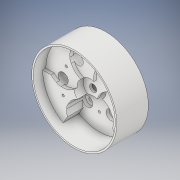
# Autodesk Inventor part: Base
Saved by Autodesk Inventor 2017 SP1 (Build 210196100, 196)
## iProperties
Created: 2017-09-22
Part Number: Base
Material: ABS Plastic
Document SubType Name: Modeling
Designer: Zach
Density: 1.06 g/cm^3
Appearance: CR White
Author: Zach
Autodesk Inventor part; units mm, degrees
ref_plane "YZ Plane" through (0, 0, 0) normal (1, 0, 0) x (0, 1, 0)
ref_plane "XZ Plane" through (0, 0, 0) normal (0, 1, 0) x (-1, 0, 0)
ref_plane "XY Plane" through (0, 0, 0) normal (0, 0, 1) x (1, 0, 0)
sketch "Sketch1" plane through (0, 0, 0) normal (0, 0, 1) x (1, 0, 0)
  circle A0 centre (0, 0) radius 54
  dimension "d0" = 108
  constraints: 1 centre point, 1 coincident
  measures "d0" diameter of A0
extrude "Extrusion1" add sketch "Sketch1" along normal blind 37
sketch "Sketch2" plane through (0, 0, 37) normal (0, 0, 1) x (1, 0, 0)
  circle A0 centre (0, 0) radius 54 projected
  circle A1 centre (0, 0) radius 52
  dimension "d3" = 2
  constraints: 1 centre point
  measures "d3" radial gap between concentric circles of A0 A1
extrude "Extrusion2" cut sketch "Sketch2" against normal blind 29 contours A1
sketch "Sketch3" plane through (0, 0, 8) normal (0, 0, 1) x (1, 0, 0)
  circle A0 centre (0, 0) radius 11
  dimension "d6" = 22
  constraints: 1 centre point, 1 coincident
  measures "d6" diameter of A0
extrude "Extrusion3" cut sketch "Sketch3" against normal through all
sketch "Sketch4" plane through (0, 0, 8) normal (0, 0, 1) x (1, 0, 0)
  circle A0 centre (30, 0) radius 6.5
  circle A1 centre (15, 25.9808) radius 6.5
  circle A2 centre (-15, 25.9808) radius 6.5
  circle A3 centre (-30, 0) radius 6.5
  circle A4 centre (-15, -25.9808) radius 6.5
  circle A5 centre (15, -25.9808) radius 6.5
  point P0 (0, 0)
  dimension "d9" = 13
  dimension "d10" = 30
  dimension "d13" = 360
  constraints: 6 centre point, 1 horizontal alignment, 13 other
  measures "d9" diameter of A0
  measures "d10" distance of point (0, 0) A0.centre
extrude "Extrusion4" cut sketch "Sketch4" against normal blind 4
sketch "Sketch5" plane through (0, 0, 8) normal (0, 0, 1) x (1, 0, 0)
  circle A0 centre (-15, -25.9808) radius 6.5 construction
  circle A1 centre (-15, 25.9808) radius 6.5 construction
  circle A2 centre (30, 0) radius 6.5 construction
  circle A3 centre (15, 25.9808) radius 6.5 construction
  circle A4 centre (-30, 0) radius 6.5 construction
  circle A5 centre (15, -25.9808) radius 6.5 construction
  circle A6 centre (0, 0) radius 11 construction
  circle A7 centre (0, 0) radius 52 construction
  circle A8 centre (30, 0) radius 2.5
  circle A9 centre (15, 25.9808) radius 2.5
  circle A10 centre (-15, 25.9808) radius 2.5
  circle A11 centre (-30, 0) radius 2.5
  circle A12 centre (-15, -25.9808) radius 2.5
  circle A13 centre (15, -25.9808) radius 2.5
  dimension "d17" = 5
  dimension "d20" = 360
  constraints: 14 centre point, 6 coincident, 19 other
  measures "d17" diameter of A8
extrude "Extrusion5" cut sketch "Sketch5" against normal through all
sketch "Sketch6" plane through (0, 0, 8) normal (0, 0, 1) x (1, 0, 0)
  circle A0 centre (0, 30) radius 1.5
  circle A1 centre (-25.9808, 15) radius 1.5
  circle A2 centre (-25.9808, -15) radius 1.5
  circle A3 centre (0, -30) radius 1.5
  circle A4 centre (25.9808, -15) radius 1.5
  circle A5 centre (25.9808, 15) radius 1.5
  point P0 (0, 0)
  dimension "d24" = 3
  dimension "d25" = 30
  dimension "d28" = 360
  constraints: 6 centre point, 1 vertical alignment, 13 other
  measures "d24" diameter of A0
  measures "d25" distance of point (0, 0) A0.centre
extrude "Extrusion6" cut sketch "Sketch6" against normal through all
sketch "Sketch7" plane through (0, 0, 8) normal (0, 0, 1) x (1, 0, 0)
  circle A0 centre (25.9808, -15) radius 1.5 projected
  circle A1 centre (25.9808, -15) radius 1.5 projected
  circle A2 centre (25.9808, -15) radius 8.5 construction
  circle A3 centre (25.9808, 15) radius 1.5 construction
  circle A4 centre (25.9808, 15) radius 21.5 construction
  circle A5 centre (0, -30) radius 1.5 construction
  circle A6 centre (0, -30) radius 21.5 construction
  circle A7 centre (0, 0) radius 12.5 construction
  arc A8 (18.6195, -19.25) -> (7.6315, -9.9) centre (0, -30) ccw
  arc A9 (7.6315, -9.9) -> (12.3894, -1.6591) centre (0, 0) ccw
  circle A10 centre (30, 0) radius 6.5 construction
  circle A11 centre (15, -25.9808) radius 6.5 construction
  circle A12 centre (25.9808, -15) radius 21.5 construction
  arc A13 (19.7818, -21.578) -> (18.6195, -19.25) centre (0, -30) ccw
  arc A14 (21.3425, -27.4028) -> (19.7818, -21.578) centre (15, -25.9808) ccw
  arc A15 (20.6918, -35.8393) -> (21.3425, -27.4028) centre (0, -30) ccw
  line L0 (0, 0) -> (52, 0) construction
  circle A16 centre (0, 0) radius 52 construction
  line L1 (0, 0) -> (26, -45.0333) construction
  line L2 (41.3837, 0) -> (52, 0)
  line L3 (20.6918, -35.8393) -> (26, -45.0333)
  arc A17 (26, -45.0333) -> (52, 0) centre (0, 0) ccw
  arc A18 (12.3894, -1.6591) -> (12.3894, 1.6591) centre (0, 0) ccw
  arc A19 (28.578, 6.3425) -> (12.3894, 1.6591) centre (25.9808, -15) ccw
  arc A20 (28.578, 6.3425) -> (28.578, -6.3425) centre (30, 0) ccw
  arc A21 (28.578, -6.3425) -> (34.4028, -4.7818) centre (30, 0) ccw
  arc A22 (34.4028, -4.7818) -> (34.4028, 4.7818) centre (30, 0) ccw
  arc A23 (41.3837, 0) -> (34.4028, 4.7818) centre (25.9808, -15) ccw
  point P0 (25.9808, -6.5)
  dimension "d32" = 17
  dimension "d57" = 43
  dimension "d58" = 43
  dimension "d59" = 25
  dimension "d60" = 43
  constraints: 52 point on circle, 17 centre point, 12 concentric, 8 end point, 5 coincident, 1 horizontal, 1 point on line
  measures "d32" diameter of A2
  measures "d57" diameter of A4
  measures "d58" diameter of A6
  measures "d59" diameter of A7
  measures "d60" diameter of A12
extrude "Extrusion7" add sketch "Sketch7" along normal blind 4
sketch "Sketch8" plane through (0, 0, 8) normal (0, 0, 1) x (1, 0, 0)
  circle A0 centre (25.9808, 15) radius 1.5
  circle A1 centre (25.9808, 15) radius 8.5 construction
  circle A2 centre (25.9808, -15) radius 21.5 construction
  circle A3 centre (0, 0) radius 12.5 construction
  line L0 (0, 0) -> (26, 45.0333) construction
  arc A4 (52, 0) -> (26, -45.0333) centre (0, 0) ccw construction
  line L1 (0, 0) -> (52, 0) construction
  circle A5 centre (15, 25.9808) radius 2.5 construction
  circle A6 centre (0, 30) radius 1.5 construction
  circle A7 centre (25.9808, -15) radius 1.5 construction
  circle A8 centre (30, 0) radius 2.5 construction
  arc A9 (12.3894, 1.6591) -> (7.6315, 9.9) centre (0, 0) ccw
  circle A10 centre (15, 25.9808) radius 6.5 construction
  arc A11 (34.4028, 4.7818) -> (28.578, 6.3425) centre (30, 0) ccw construction
  circle A12 centre (30, 0) radius 6.5
  arc A13 (28.578, 6.3425) -> (12.3894, 1.6591) centre (25.9808, -15) ccw
  arc A14 (34.4028, 4.7818) -> (28.578, 6.3425) centre (30, 0) ccw
  arc A15 (41.3837, 0) -> (34.4028, 4.7818) centre (25.9808, -15) ccw
  line L2 (41.3837, 0) -> (52, 0)
  line L3 (20.6918, 35.8393) -> (26, 45.0333)
  arc A16 (52, 0) -> (26, 45.0333) centre (0, 0) ccw
  circle A17 centre (25.9808, 15) radius 21.5 construction
  circle A18 centre (0, 30) radius 1.5 projected
  circle A19 centre (0, 30) radius 21.5 construction
  circle A20 centre (15, 25.9808) radius 6.5 projected
  arc A21 (20.6918, 35.8393) -> (13.0602, 32.1846) centre (25.9808, 15) ccw
  arc A22 (13.0602, 32.1846) -> (8.7962, 27.9205) centre (15, 25.9808) ccw
  arc A23 (8.7962, 27.9205) -> (4.7579, 11.5591) centre (25.9808, 15) ccw
  arc A24 (7.6315, 9.9) -> (4.7579, 11.5591) centre (0, 0) ccw
  point P0 (18.6195, 19.25)
  point P1 (19.7818, 21.578)
  point P2 (21.3425, 27.4028)
  point P3 (28.578, -6.3425)
  point P4 (34.4028, -4.7818)
  dimension "d35" = 17
  dimension "d61" = 43
  dimension "d63" = 25
  dimension "d68" = 43
  dimension "d69" = 43
  constraints: 40 point on circle, 22 centre point, 8 end point, 7 concentric, 5 coincident, 4 point on line, 1 horizontal, 3 other
  measures "d61" diameter of A2
  measures "d63" diameter of A3
  measures "d68" diameter of A17
  measures "d69" diameter of A19
extrude "Extrusion8" add sketch "Sketch8" along normal blind 8 contours A9 A24 A23 A20 A21 L3 A16 L2 A15 A12 A13
sketch "Sketch9" plane through (0, 0, 8) normal (0, 0, 1) x (1, 0, 0)
  circle A0 centre (0, 30) radius 1.5
  circle A1 centre (0, 30) radius 8.5 construction
  arc A2 (13.0602, 32.1846) -> (8.7962, 27.9205) centre (15, 25.9808) ccw
  circle A3 centre (0, 0) radius 11
  circle A4 centre (-15, 25.9808) radius 6.5
  arc A5 (19.7818, 21.578) -> (21.3425, 27.4028) centre (15, 25.9808) ccw
  circle A6 centre (0, 0) radius 52
  line L0 (20.6918, 35.8393) -> (26, 45.0333)
  line L1 (26, 45.0333) -> (0, 0) construction
  line L2 (0, 0) -> (-26, 45.0333) construction
  circle A7 centre (-25.9808, 15) radius 1.5
  circle A8 centre (25.9808, 15) radius 1.5
  circle A9 centre (-25.9808, 15) radius 1.5
  circle A10 centre (-25.9808, 15) radius 21.5 construction
  circle A11 centre (25.9808, 15) radius 1.5
  circle A12 centre (25.9808, 15) radius 21.5 construction
  circle A13 centre (0, 0) radius 12.5 construction
  arc A14 (4.7579, 11.5591) -> (-4.7579, 11.5591) centre (0, 0) ccw
  arc A15 (8.7962, 27.9205) -> (4.7579, 11.5591) centre (25.9808, 15) ccw
  circle A16 centre (15, 25.9808) radius 6.5
  arc A17 (13.0602, 32.1846) -> (8.7962, 27.9205) centre (15, 25.9808) ccw
  arc A18 (-4.7579, 11.5591) -> (-6.25, 10.8253) centre (0, 0) ccw
  circle A19 centre (0, 30) radius 21.5 construction
  arc A20 (-6.25, 10.8253) -> (-7.6315, 9.9) centre (0, 0) ccw
  circle A21 centre (-15, 25.9808) radius 6.5
  arc A22 (-19.7818, 21.578) -> (-7.6315, 9.9) centre (0, 30) ccw
  arc A23 (-21.3425, 27.4028) -> (-19.7818, 21.578) centre (-15, 25.9808) ccw
  arc A24 (-20.6918, 35.8393) -> (-21.3425, 27.4028) centre (0, 30) ccw
  line L3 (-20.6918, 35.8393) -> (-26, 45.0333)
  arc A25 (20.6918, 35.8393) -> (13.0602, 32.1846) centre (25.9808, 15) ccw
  arc A26 (26, 45.0333) -> (26, -45.0333) centre (0, 0) ccw construction
  arc A27 (26, 45.0333) -> (-26, 45.0333) centre (0, 0) ccw construction
  line L4 (20.6918, 35.8393) -> (26, 45.0333)
  arc A28 (26, 45.0333) -> (-26, 45.0333) centre (0, 0) ccw
  dimension "d38" = 17
  dimension "d64" = 43
  dimension "d65" = 43
  dimension "d66" = 25
  dimension "d67" = 43
  constraints: 44 point on circle, 27 centre point, 10 end point, 9 concentric, 5 coincident, 2 point on line, 1 collinear, 7 other
  measures "d38" diameter of A1
  measures "d64" diameter of A10
  measures "d65" diameter of A12
  measures "d66" diameter of A13
  measures "d67" diameter of A19
extrude "Extrusion9" add sketch "Sketch9" along normal blind 12 contours A2 A15 A14 A18 A20 A22 A4 A24 L3 A6 L0 A25
sketch "Sketch10" plane through (0, 0, 8) normal (0, 0, 1) x (1, 0, 0)
  circle A0 centre (-25.9808, 15) radius 1.5 projected
  circle A1 centre (-25.9808, 15) radius 8.5 construction
  circle A2 centre (0, 30) radius 1.5 projected
  arc A3 (-19.7818, 21.578) -> (-21.3425, 27.4028) centre (-15, 25.9808) ccw projected
  arc A4 (-21.3425, 27.4028) -> (-19.7818, 21.578) centre (-15, 25.9808) ccw projected
  circle A5 centre (-30, 0) radius 6.5 projected
  circle A6 centre (-25.9808, -15) radius 1.5 projected
  line L0 (0, 0) -> (-52, 0) construction
  arc A7 (-26, 45.0333) -> (26, -45.0333) centre (0, 0) ccw projected
  circle A8 centre (-25.9808, -15) radius 1.5 projected
  circle A9 centre (-25.9808, -15) radius 21.5 construction
  circle A10 centre (-25.9808, 15) radius 21.5 construction
  circle A11 centre (0, 30) radius 21.5 construction
  circle A12 centre (0, 0) radius 12.5 construction
  arc A13 (-19.7818, 21.578) -> (-7.6315, 9.9) centre (0, 30) ccw projected
  arc A14 (-7.6315, 9.9) -> (-12.3894, -1.6591) centre (0, 0) ccw
  arc A15 (-28.578, -6.3425) -> (-12.3894, -1.6591) centre (-25.9808, 15) ccw
  circle A16 centre (-30, 0) radius 6.5 projected
  arc A17 (-34.4028, -4.7818) -> (-28.578, -6.3425) centre (-30, 0) ccw
  arc A18 (-41.3837, 0) -> (-34.4028, -4.7818) centre (-25.9808, 15) ccw
  line L1 (-41.3837, 0) -> (-52, 0)
  line L2 (-26, 45.0333) -> (-20.6918, 35.8393) projected
  arc A19 (-20.6918, 35.8393) -> (-21.3425, 27.4028) centre (0, 30) ccw projected
  arc A20 (-19.7818, 21.578) -> (-7.6315, 9.9) centre (0, 30) ccw projected
  arc A21 (-26, 45.0333) -> (-52, 0) centre (0, 0) ccw
  dimension "d70" = 43
  dimension "d73" = 25
  dimension "d41" = 17
  dimension "d71" = 43
  dimension "d72" = 43
  constraints: 15 point on circle, 8 centre point, 5 coincident, 4 end point, 3 concentric, 1 horizontal, 12 other
  measures "d41" diameter of A1
  measures "d71" diameter of A10
  measures "d72" diameter of A11
extrude "Extrusion10" add sketch "Sketch10" along normal blind 16 contours A13 A14 A15 A5 A18 L1 A7 L2 A19 A4
sketch "Sketch11" plane through (0, 0, 8) normal (0, 0, 1) x (1, 0, 0)
  circle A0 centre (-25.9808, -15) radius 1.5 projected
  circle A1 centre (-25.9808, -15) radius 8.5 construction
  circle A2 centre (0, -30) radius 1.5 projected
  arc A3 (-34.4028, -4.7818) -> (-28.578, -6.3425) centre (-30, 0) ccw projected
  arc A4 (-28.578, -6.3425) -> (-12.3894, -1.6591) centre (-25.9808, 15) ccw projected
  arc A5 (-41.3837, 0) -> (-34.4028, -4.7818) centre (-25.9808, 15) ccw projected
  line L0 (-52, 0) -> (-41.3837, 0) projected
  circle A6 centre (0, 0) radius 52 projected
  circle A7 centre (-15, -25.9808) radius 6.5 projected
  circle A8 centre (0, -30) radius 21.5 construction
  circle A9 centre (0, 0) radius 12.5 construction
  line L1 (0, 0) -> (-26, -45.0333) construction
  arc A10 (-12.3894, -1.6591) -> (-7.6315, -9.9) centre (0, 0) ccw
  circle A11 centre (-15, -25.9808) radius 6.5 projected
  arc A12 (-7.6315, -9.9) -> (-19.7818, -21.578) centre (0, -30) ccw
  arc A13 (-19.7818, -21.578) -> (-21.3425, -27.4028) centre (-15, -25.9808) ccw
  arc A14 (-21.3425, -27.4028) -> (-20.6918, -35.8393) centre (0, -30) ccw
  line L2 (-20.6918, -35.8393) -> (-26, -45.0333)
  arc A15 (-52, 0) -> (-26, -45.0333) centre (0, 0) ccw
  dimension "d75" = 25
  dimension "d44" = 17
  dimension "d74" = 43
  constraints: 15 point on circle, 7 centre point, 4 concentric, 4 end point, 3 coincident, 2 point on line, 1 collinear, 9 other
  measures "d44" diameter of A1
  measures "d74" diameter of A8
extrude "Extrusion11" add sketch "Sketch11" along normal blind 20 contours A3 A4 A10 A12 A7 A14 L2 A6 L0 A5 picked at (-29.3886, -25.1687)
sketch "Sketch15" plane through (0, 0, 37) normal (0, 0, 1) x (1, 0, 0)
  circle A0 centre (0, 0) radius 52 projected
  circle A1 centre (0, 0) radius 54 projected
extrude "Extrusion15" add sketch "Sketch15" along normal blind 3
sketch "Sketch17" plane through (0, 0, 8) normal (0, 0, 1) x (1, 0, 0)
  circle A0 centre (0, 0) radius 11 projected
  circle A1 centre (0, 0) radius 4.5
  dimension "d76" = 9
  constraints: 1 centre point, 1 coincident
  measures "d76" diameter of A1
extrude "Extrusion16" add sketch "Sketch17" against normal blind 1
sketch "Sketch19" plane through (0, 0, 12) normal (0, 0, 1) x (1, 0, 0)
  circle A0 centre (0, 0) radius 12.5
  circle A1 centre (0, 0) radius 4.5 projected
  dimension "d80" = 25
  constraints: 1 centre point, 1 coincident
  measures "d80" diameter of A0
extrude "Extrusion17" add sketch "Sketch19" along normal blind 4
sketch "Sketch20" plane through (0, 0, 12) normal (0, 0, 1) x (1, 0, 0)
  circle A0 centre (25.9808, -15) radius 1.5 projected
  circle A1 centre (25.9808, -15) radius 21.5
  arc A2 (28.578, 6.3425) -> (12.3894, 1.6591) centre (25.9808, -15) ccw projected
  point P0 (0, 0)
  constraints: 1 coincident, 4 other
extrude "Extrusion18" cut sketch "Sketch20" along normal blind 4
sketch "Sketch21" plane through (0, 0, 8) normal (0, 0, 1) x (1, 0, 0)
  arc A0 (12.3894, 1.6591) -> (-7.6315, -9.9) centre (0, 0) ccw projected
  line L0 (-21.2785, -24.2984) -> (-7.6315, -9.9)
  arc A1 (-11.8566, 3.9587) -> (-7.6315, -9.9) centre (0, 0) ccw
  arc A2 (-19.7818, -21.578) -> (-21.3425, -27.4028) centre (-15, -25.9808) ccw projected
  arc A3 (-11.5923, 4.6764) -> (-21.2785, -24.2984) centre (221.4767, -89.3445) ccw
  point P0 (0, 0)
  constraints: 7 point on circle, 2 centre point, 2 end point, 2 tangent, 1 concentric
extrude "Extrusion19" cut sketch "Sketch21" along normal blind 4
sketch "Sketch24" plane through (0, 0, 8) normal (0, 0, 1) x (1, 0, 0)
  circle A0 centre (0, 0) radius 4.5 projected
  circle A1 centre (0, 0) radius 12.5
  dimension "d89" = 25
  constraints: 1 centre point, 1 coincident
  measures "d89" diameter of A1
extrude "Extrusion21" cut sketch "Sketch24" along normal blind 5
sketch "Sketch25" plane through (0, 0, 8) normal (0, 0, 1) x (1, 0, 0)
  arc A0 (-11.5923, 4.6764) -> (-21.2785, -24.2984) centre (221.4767, -89.3445) ccw projected
  arc A1 (-7.6315, -9.9) -> (-19.7818, -21.578) centre (0, -30) ccw projected
  arc A2 (-12.3894, -1.6591) -> (-7.6315, -9.9) centre (0, 0) ccw projected
  arc A3 (-11.5923, 4.6764) -> (-12.3894, -1.6591) centre (0, 0) ccw
  arc A4 (-19.7818, -21.578) -> (-21.2785, -24.2984) centre (-15, -25.9808) ccw
  circle A5 centre (-15, -25.9808) radius 6.5 projected
  point P0 (0, 0)
  constraints: 5 point on circle, 3 concentric, 2 centre point
extrude "Extrusion22" cut sketch "Sketch25" along normal blind 5 contours A3 A2 A1 A4 A0
sketch "Sketch26" plane through (0, 0, 8) normal (0, 0, 1) x (1, 0, 0)
  circle A0 centre (0, -30) radius 1.5 projected
  circle A1 centre (0, -30) radius 21.5
  point P0 (0, 0)
  dimension "d94" = 43
  constraints: 1 centre point, 1 coincident
  measures "d94" diameter of A1
extrude "Extrusion23" cut sketch "Sketch26" along normal through all
body "Solid1"
